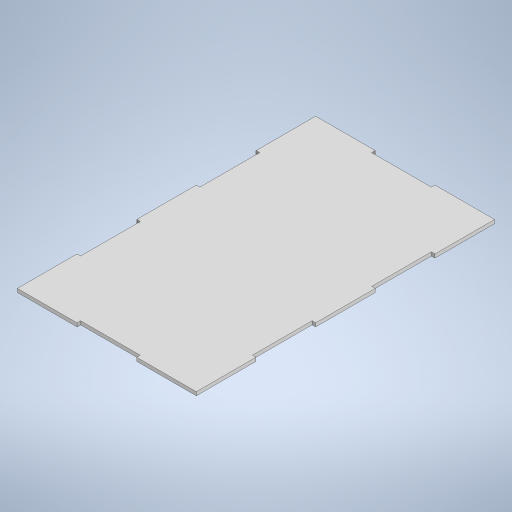
# Autodesk Inventor part: Alas Bawah
Saved by Autodesk Inventor 2024 (Build 280153000, 153)
## iProperties
Created: 2023-07-10
Part Number: Alas Bawah
Material: Generic
Document SubType Name: Modeling
Designer: Asus
Density: 1 g/cm^3
Appearance: Default
Author: Asus
Autodesk Inventor part; units mm, degrees
ref_plane "YZ Plane" through (0, 0, 0) normal (1, 0, 0) x (0, 1, 0)
ref_plane "XZ Plane" through (0, 0, 0) normal (0, 1, 0) x (-1, 0, 0)
ref_plane "XY Plane" through (0, 0, 0) normal (0, 0, 1) x (1, 0, 0)
sketch "Sketch2" plane through (0, 0, 0) normal (0, 1, 0) x (-1, 0, 0)
  line L0 (0, 0) -> (0, -50)
  line L1 (0, -50) -> (3, -50)
  line L2 (3, -50) -> (3, -100)
  line L3 (3, -100) -> (0, -100)
  line L4 (0, -100) -> (0, -150)
  line L5 (0, -150) -> (3, -150)
  line L6 (3, -150) -> (3, -200)
  line L7 (3, -200) -> (0, -200)
  line L8 (0, -200) -> (0, -250)
  line L9 (0, -250) -> (50, -250)
  line L10 (50, -250) -> (50, -247)
  line L11 (50, -247) -> (100, -247)
  line L12 (100, -247) -> (100, -250)
  line L13 (100, -250) -> (150, -250)
  line L14 (150, -250) -> (150, -200)
  line L15 (150, -200) -> (147, -200)
  line L16 (147, -200) -> (147, -150)
  line L17 (147, -150) -> (150, -150)
  line L18 (150, -150) -> (150, -100)
  line L19 (150, -100) -> (147, -100)
  line L20 (147, -100) -> (147, -50)
  line L21 (147, -50) -> (150, -50)
  line L22 (150, -50) -> (150, 0)
  line L23 (150, 0) -> (100, 0)
  line L24 (100, 0) -> (100, -3)
  line L25 (100, -3) -> (50, -3)
  line L26 (50, -3) -> (50, 0)
  line L27 (50, 0) -> (0, 0)
  dimension "d2" = 50
  dimension "d3" = 3
  dimension "d4" = 50
  dimension "d5" = 3
  dimension "d6" = 50
  dimension "d7" = 50
  dimension "d8" = 50
  dimension "d9" = 50
  dimension "d10" = 3
  dimension "d11" = 50
  dimension "d12" = 50
  dimension "d13" = 50
  dimension "d14" = 3
  dimension "d15" = 50
  dimension "d16" = 50
  dimension "d17" = 50
  dimension "d18" = 50
  dimension "d19" = 3
  dimension "d20" = 50
  constraints: 56 end point, 16 perpendicular, 16 point on line, 2 vertical
  measures "d2" distance of L0.start L0.end
  measures "d3" distance of L0.end L1.end
  measures "d4" distance of L1.end L2.end
  measures "d5" distance of L2.end L3.end
  measures "d6" distance of L3.end L4.end
  measures "d7" distance of L5.end L6.end
  measures "d8" distance of L7.end L8.end
  measures "d9" distance of L8.end L9.end
  measures "d10" distance of L9.end L10.end
  measures "d11" distance of L10.end L11.end
  measures "d12" distance of L12.end L13.end
  measures "d13" distance of L13.end L14.end
  measures "d14" distance of L14.end L15.end
  measures "d15" distance of L15.end L16.end
  measures "d16" distance of L17.end L18.end
  measures "d17" distance of L19.end L20.end
  measures "d18" distance of L22.end L23.end
  measures "d19" distance of L23.end L24.end
  measures "d20" distance of L24.end L25.end
extrude "Extrusion1" add sketch "Sketch2" along normal blind 3
body "Solid1"
